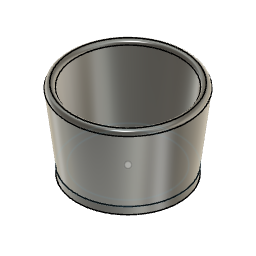
nob_cover (Autodesk Fusion 360 design; units mm, degrees)
Autodesk Fusion 360 part; units mm, degrees
sketch "Sketch1" plane through (0, 0, 0) normal (0, 0, 1) x (1, 0, 0)
  circle A0 centre (18.128, 18.245) radius 25.47
  circle A1 centre (18.128, 18.245) radius 21.47
  dimension "d5" = 50.94
  dimension "d6" = 42.94
  constraint concentric A0 A1
  measures "d5" diameter of A0
  measures "d6" diameter of A1
sketch "Sketch2" plane through (0, 0, 0) normal (0, 0, 1) x (1, 0, 0)
ref_plane "WorkPlane1" through (0, 0, 35.41) normal (0, 0, 1) x (1, 0, 0)
sketch "Sketch3" plane through (0, 0, 35.41) normal (0, 0, 1) x (1, 0, 0)
  circle A0 centre (18.128, 18.245) radius 29.87
  circle A1 centre (18.128, 18.245) radius 25.87
  point P0 (18.128, 18.245)
  dimension "d8" = 59.74
  dimension "d9" = 51.74
  constraint coincident P0 A0.centre
  measures "d8" diameter of A0
  measures "d9" diameter of A1
loft "Loft1" add profiles "Sketch3", "Sketch1" section 1 section 2 makes body 1
sketch "Sketch4" plane through (0, 0, 35.41) normal (0, 0, 1) x (-1, 0, 0)
  circle A0 centre (-18.128, -18.245) radius 29.87
  circle A1 centre (-18.128, -18.245) radius 25.87
  dimension "d10" = 51.74
  constraint concentric A0 A1
  measures "d10" diameter of A1
sketch "Sketch5" plane through (0, 0, 35.41) normal (0, 0, 1) x (-1, 0, 0)
  circle A0 centre (-18.128, -18.245) radius 29.87
sketch "Sketch6" plane through (0, 0, 35.41) normal (0, 0, 1) x (1, 0, 0)
  circle A0 centre (18.128, 18.245) radius 25.87
  point P0 (18.128, 18.245)
  dimension "d15" = 51.74
  constraint coincident P0 A0.centre
  measures "d15" diameter of A0
loft "Loft2" cut profiles "Sketch1", "Sketch6" section 1 contours A1 section 2 bodies 1
extrude "Extrude2" add sketch "Sketch1" against normal blind 3.541 contours A0 | A1 bodies 1
copy_body "Body->Comp2" bodies 1 removing the originals makes body 2 in component "Component"
fillet "Fillet1" radius 2 1 faces at (46.4571, 15.4758, 35.41) on bodies 2 in component "Component"
component "Component" placed x (1, 0, 0) y (0, 1, 0) z (0, 0, 1) at (0, 0, 0)
equation "nob_widest_rad = 25.87 mm"
equation "nob_narrowest_rad = 21.47 mm"
equation "nob_len = 35.41 mm"
equation "nob_cover_thickness = 4 mm"
equation "d5 = ( nob_narrowest_rad + nob_cover_thickness ) * 2"
equation "d6 = nob_narrowest_rad * 2"
equation "d7 = nob_len"
equation "d8 = ( nob_widest_rad + nob_cover_thickness ) * 2"
equation "d9 = nob_widest_rad * 2"
equation "d10 = nob_widest_rad * 2"
equation "d15 = ( nob_widest_rad ) * 2"
equation "d16 = -nob_len * 0.1"
